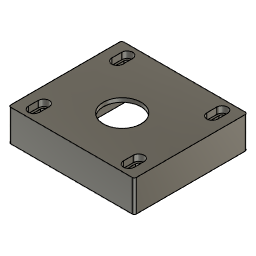
servo motor spindle drive (Autodesk Fusion 360 archive; units mm, degrees)
design "pulley cover"
Autodesk Fusion 360 part; units mm, degrees
note: some values were not read from the file. Chosen so that the rebuilt part matches the saved one: a direction.
sketch "Sketch1" plane through (0, 0, 0) normal (0, 0, 1) x (1, 0, 0)
  line L0 (63.5, -57.15) -> (-63.5, -57.15)
  line L1 (-63.5, -57.15) -> (-63.5, 57.15)
  line L2 (-63.5, 57.15) -> (63.5, 57.15)
  line L3 (63.5, 57.15) -> (63.5, -57.15)
  line L4 (63.5, -57.15) -> (-63.5, 57.15) construction
  line L5 (-63.5, -57.15) -> (63.5, 57.15) construction
  dimension "d1" = 127
  dimension "d2" = 114.3
  constraint perpendicular L0 L1
  constraint parallel L0 L2
  constraint parallel L1 L3
  constraint horizontal L0
  constraint coincident L4 origin
  constraint coincident L5 origin
  measures "d1" distance of L1.end L2.end
  measures "d2" distance of L0.end L1.end
extrude "Extrude1" add sketch "Sketch1" along normal blind 32
sketch "Sketch2" plane through (0, 0, 0) normal (0, 0, -1) x (1, 0, 0)
  line L0 (-63.5, -57.15) -> (63.5, -57.15)
  line L1 (63.5, -57.15) -> (63.5, 57.15)
  line L2 (63.5, 57.15) -> (-63.5, 57.15)
  line L3 (-63.5, 57.15) -> (-63.5, -57.15)
  line L4 (-40, 5.85) -> (40, 5.85) construction
  line L5 (40, 5.85) -> (40, -57.15)
  line L6 (40, -57.15) -> (-40, -57.15)
  line L7 (-40, -57.15) -> (-40, 5.85)
  line L8 (0, 0) -> (0, 57.15) construction
  arc A0 (40, 5.85) -> (-40, 5.85) centre (0, 5.85) ccw
  arc A1 (-40, 5.85) -> (40, 5.85) centre (0, 5.85) ccw construction
  dimension "d5" = 40
  dimension "d20" = 63
  constraint horizontal L4
  constraint vertical L5
  constraint horizontal L6
  constraint vertical L7
  constraint coincident L0 L5.end
  constraint coincident L8.start origin
  constraint midpoint L2 L8.end
  constraint coincident A0.centre L8
  constraint midpoint A0.centre L4
  constraint concentric A0 A1
  measures "d5" radius of A0
  measures "d20" distance of L0 A0.centre
extrude "Extrude2" cut sketch "Sketch2" against normal blind 28 contours L0 L5 L6 L7 A0
sketch "Sketch3" plane through (0, 0, 28) normal (0, 0, -1) x (1, 0, 0)
  line L0 (40, -57.15) -> (40, 5.85)
  arc A0 (40, 5.85) -> (-40, 5.85) centre (0, 5.85) ccw
  line L1 (-40, 5.85) -> (-40, -57.15)
  line L2 (-40, -57.15) -> (40, -57.15)
  circle A1 centre (0, 5.85) radius 19.05
  dimension "d9" = 38.1
  constraint concentric A0 A1
  measures "d9" diameter of A1
extrude "Extrude3" cut sketch "Sketch3" against normal through all contours A1
fillet "Fillet1" radius 2 6 edges at (-63.5, 57.15, 16) (63.5, 57.15, 16) (63.5, -57.15, 16) (-63.5, -57.15, 16) (-40, 57.15, 14) (40, 57.15, 14)
sketch "Sketch4" plane through (0, 0, 32) normal (0, 0, 1) x (-1, 0, 0)
  circle A0 centre (0, 5.85) radius 19.05
  arc A1 (-63.5, -55.15) -> (-61.5, -57.15) centre (-61.5, -55.15) ccw
  line L0 (-61.5, -57.15) -> (61.5, -57.15)
  arc A2 (61.5, -57.15) -> (63.5, -55.15) centre (61.5, -55.15) ccw
  line L1 (63.5, -55.15) -> (63.5, 55.15)
  arc A3 (63.5, 55.15) -> (61.5, 57.15) centre (61.5, 55.15) ccw
  line L2 (61.5, 57.15) -> (-61.5, 57.15)
  arc A4 (-61.5, 57.15) -> (-63.5, 55.15) centre (-61.5, 55.15) ccw
  line L3 (-63.5, 55.15) -> (-63.5, -55.15)
  line L4 (44.7, -37.15) -> (44.7, -47.15)
  arc A5 (44.7, -47.15) -> (51.3, -47.15) centre (48, -47.15) ccw
  line L5 (51.3, -47.15) -> (51.3, -37.15)
  arc A6 (51.3, -37.15) -> (44.7, -37.15) centre (48, -37.15) ccw
  line L6 (48, -37.15) -> (48, -47.15) construction
  line L7 (53.5, -47.15) -> (53.5, -37.15)
  arc A7 (53.5, -37.15) -> (42.5, -37.15) centre (48, -37.15) ccw
  line L8 (42.5, -37.15) -> (42.5, -47.15)
  arc A8 (42.5, -47.15) -> (53.5, -47.15) centre (48, -47.15) ccw
  line L9 (48, -47.15) -> (48, -37.15) construction
  line L10 (0, -57.15) -> (0, 57.15) construction
  line L11 (63.5, 0) -> (-63.5, 0) construction
  arc A9 (-53.5, -47.15) -> (-42.5, -47.15) centre (-48, -47.15) ccw
  arc A10 (-44.7, -37.15) -> (-51.3, -37.15) centre (-48, -37.15) ccw
  line L12 (-53.5, -47.15) -> (-53.5, -37.15)
  line L13 (-48, -47.15) -> (-48, -37.15) construction
  arc A11 (-42.5, -37.15) -> (-53.5, -37.15) centre (-48, -37.15) ccw
  line L14 (-48, -37.15) -> (-48, -47.15) construction
  arc A12 (-51.3, -47.15) -> (-44.7, -47.15) centre (-48, -47.15) ccw
  line L15 (-51.3, -47.15) -> (-51.3, -37.15)
  line L16 (-42.5, -37.15) -> (-42.5, -47.15)
  line L17 (-44.7, -37.15) -> (-44.7, -47.15)
  line L18 (44.7, 37.15) -> (44.7, 47.15)
  arc A13 (42.5, 37.15) -> (53.5, 37.15) centre (48, 37.15) ccw
  line L19 (53.5, 47.15) -> (53.5, 37.15)
  line L20 (51.3, 47.15) -> (51.3, 37.15)
  arc A14 (44.7, 37.15) -> (51.3, 37.15) centre (48, 37.15) ccw
  arc A15 (53.5, 47.15) -> (42.5, 47.15) centre (48, 47.15) ccw
  line L21 (48, 47.15) -> (48, 37.15) construction
  arc A16 (51.3, 47.15) -> (44.7, 47.15) centre (48, 47.15) ccw
  line L22 (48, 37.15) -> (48, 47.15) construction
  line L23 (42.5, 37.15) -> (42.5, 47.15)
  arc A17 (-53.5, 37.15) -> (-42.5, 37.15) centre (-48, 37.15) ccw
  line L24 (-44.7, 37.15) -> (-44.7, 47.15)
  arc A18 (-42.5, 47.15) -> (-53.5, 47.15) centre (-48, 47.15) ccw
  line L25 (-42.5, 37.15) -> (-42.5, 47.15)
  line L26 (-48, 47.15) -> (-48, 37.15) construction
  arc A19 (-44.7, 47.15) -> (-51.3, 47.15) centre (-48, 47.15) ccw
  line L27 (-51.3, 47.15) -> (-51.3, 37.15)
  line L28 (-53.5, 47.15) -> (-53.5, 37.15)
  line L29 (-48, 37.15) -> (-48, 47.15) construction
  arc A20 (-51.3, 37.15) -> (-44.7, 37.15) centre (-48, 37.15) ccw
  point P0 (48, -42.15)
  point P1 (-48, -42.15)
  point P2 (48, 42.15)
  point P3 (-48, 42.15)
  dimension "d12" = 6.6
  dimension "d13" = 10
  dimension "d14" = 15
  dimension "d16" = 11
  dimension "d21" = 48
  constraint tangent L4 A5
  constraint tangent A5 L5
  constraint parallel L4 L5
  constraint tangent L5 A6
  constraint tangent L4 A6
  constraint vertical L6
  constraint midpoint L6 P0
  constraint tangent L7 A7
  constraint tangent A7 L8
  constraint parallel L7 L8
  constraint tangent L8 A8
  constraint tangent L7 A8
  constraint coincident A6.centre L6.start
  constraint parallel L6 L9
  constraint coincident A5.centre L6.end
  constraint midpoint L0 L10.start
  constraint midpoint L2 L10.end
  constraint midpoint L1 L11.start
  constraint midpoint L3 L11.end
  constraint symmetric L4.start L10 A10.start
  constraint symmetric L4.end L10 A12.end
  constraint symmetric A5.end L10 A12.start
  constraint symmetric L5.end L10 A10.end
  constraint symmetric A5 L10 A12
  constraint symmetric A6 L10 A10
  constraint symmetric P0 L10 P1
  constraint symmetric L7.start L10 A9.start
  constraint symmetric L7.end L10 L12.end
  constraint symmetric A7.end L10 A11.start
  constraint symmetric L8.end L10 A9.end
  constraint symmetric A7 L10 A11
  constraint symmetric A8 L10 A9
  constraint symmetric L4.start L11 L18.start
  constraint symmetric L4.end L11 L18.end
  constraint symmetric A5.end L11 L20.start
  constraint symmetric L5.end L11 L20.end
  constraint symmetric A5 L11 A16
  constraint symmetric A6 L11 A14
  constraint symmetric P0 L11 P2
  constraint symmetric L7.start L11 L19.start
  constraint symmetric L7.end L11 A13.end
  constraint symmetric A7.end L11 A13.start
  constraint symmetric L8.end L11 A15.end
  constraint symmetric A7 L11 A13
  constraint symmetric A8 L11 A15
  constraint symmetric L11 A10.end L27.end
  constraint symmetric L11 P1 P3
  constraint symmetric L11 A9.end A18.start
  constraint symmetric L11 A9.start A18.end
  constraint symmetric L11 L12.end A17.start
  constraint symmetric L11 A12.end L24.end
  constraint symmetric L11 A12.start A19.end
  constraint symmetric L11 A11.start A17.end
  constraint symmetric L11 A10.start L24.start
  constraint symmetric L11 A9 A18
  constraint symmetric L11 A10 A20
  constraint symmetric L11 A11 A17
  constraint symmetric L11 A12 A19
  measures "d12" diameter of A5
  measures "d13" distance of A6.centre A5.centre
  measures "d14" distance of L0 P0
  measures "d16" diameter of A7
  measures "d21" distance of L6 L10
extrude "Extrude4" cut sketch "Sketch4" against normal through all contours L4 A5 L5 A6 | A10 A12 L15 L17 | L18 L20 A14 A16 | L24 A19 L27 A20
extrude "Extrude5" cut sketch "Sketch4" against normal blind 6.5 contours L7 A7 L8 A8 | A9 L12 A11 L16 | A13 L19 A15 L23 | A17 A18 L25 L28

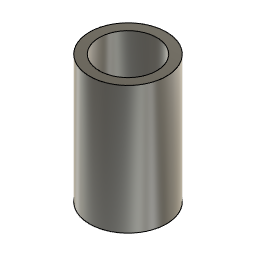
design "pivot sleeve"
Autodesk Fusion 360 part; units mm, degrees
sketch "Sketch1" plane through (0, 0, 0) normal (0, 0, 1) x (1, 0, 0)
  circle A0 centre (0, 0) radius 6
  circle A1 centre (0, 0) radius 4.5
  dimension "d1" = 12
  dimension "d2" = 9
  constraint coincident A0.centre A1.centre
  constraint concentric A0 A1
  measures "d1" diameter of A0
  measures "d2" diameter of A1
extrude "Extrude1" add sketch "Sketch1" along normal blind 20
